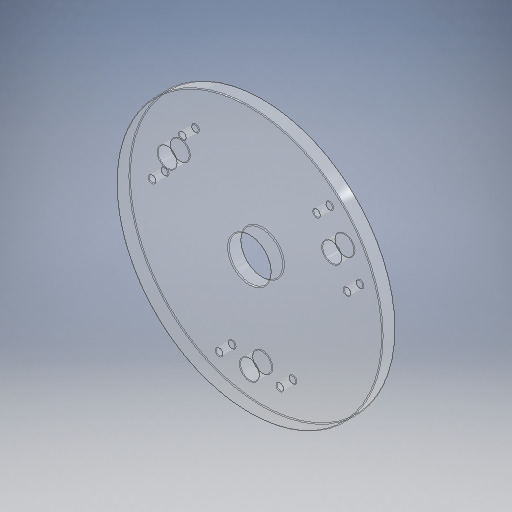
# Autodesk Inventor part: Topo
Saved by Autodesk Inventor 2025.1 (Build 291241020, 241B)
## iProperties
Created: 2025-05-02
Part Number: Topo
Material: Generic
Document SubType Name: Modeling
Designer: Nelson
Density: 1 g/cm^3
Appearance: Polycarbonate - Clear
Author: Nelson
Autodesk Inventor part; units mm, degrees
ref_plane "YZ Plane" through (0, 0, 0) normal (1, 0, 0) x (0, 1, 0)
ref_plane "XZ Plane" through (0, 0, 0) normal (0, 1, 0) x (-1, 0, 0)
ref_plane "XY Plane" through (0, 0, 0) normal (0, 0, 1) x (1, 0, 0)
sketch "Sketch1" plane through (0, 0, 0) normal (0, 0, 1) x (1, 0, 0)
  circle A0 centre (0, 0) radius 70
  circle A1 centre (0, 0) radius 50 construction
  circle A2 centre (0, -50) radius 5
  line L0 (0, -50) -> (16, -50) construction
  circle A3 centre (16, -50) radius 1.75
  line L1 (0, -50) -> (-16, -50) construction
  circle A4 centre (-16, -50) radius 1.75
  circle A5 centre (35.3013, 38.8564) radius 1.75
  line L2 (43.3013, 25) -> (35.3013, 38.8564) construction
  circle A6 centre (43.3013, 25) radius 5
  line L3 (43.3013, 25) -> (51.3013, 11.1436) construction
  circle A7 centre (51.3013, 11.1436) radius 1.75
  circle A8 centre (-51.3013, 11.1436) radius 1.75
  line L4 (-43.3013, 25) -> (-51.3013, 11.1436) construction
  circle A9 centre (-43.3013, 25) radius 5
  line L5 (-43.3013, 25) -> (-35.3013, 38.8564) construction
  circle A10 centre (-35.3013, 38.8564) radius 1.75
  circle A11 centre (0, 0) radius 11
  dimension "D_F" = 100
  dimension "D_B" = 140
  dimension "Furos" = 10
  dimension "d3" = 16
  dimension "d4" = 3.5
  dimension "d5" = 16
  dimension "d6" = 3.5
  dimension "d9" = 360
  dimension "d11" = 22
  constraints: 12 end point, 11 centre point, 9 coincident, 3 point on line, 2 horizontal, 1 vertical alignment, 33 other
  measures "D_B" diameter of A0
  measures "Furos" diameter of A2
  measures "d3" distance of L0.start L0.end
  measures "d4" diameter of A3
  measures "d5" distance of L0.start L1.end
  measures "d6" diameter of A4
  measures "d11" diameter of A11
extrude "Extrusion1" add sketch "Sketch1" along normal blind 7
fillet "Fillet1" radius 0.4 2 edges at (-70, 0, 7) (-70, 0, 0)
fillet "Fillet2" radius 0.5 2 edges at (-11, 0, 0) (-11, 0, 7)
fillet "Fillet3" radius 0.3 18 edges at (33.5513, 38.8564, 7) (38.3013, 25, 7) (49.5513, 11.1436, 7) (14.25, -50, 7) (-5, -50, 7) (-17.75, -50, 7) (-53.0513, 11.1436, 7) (-48.3013, 25, 7) (-37.0513, 38.8564, 7) (-17.75, -50, 0) (-5, -50, 0) (14.25, -50, 0) (49.5513, 11.1436, 0) (38.3013, 25, 0) (33.5513, 38.8564, 0) (-37.0513, 38.8564, 0) (-48.3013, 25, 0) (-53.0513, 11.1436, 0)
body "Solid1"
